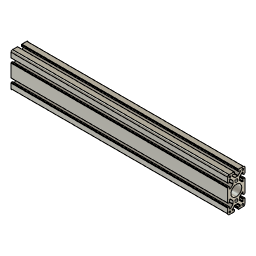
Profile 40x80 (Autodesk Fusion 360 design; units mm, degrees)
Autodesk Fusion 360 part; units mm, degrees
sketch "Sketch1" plane through (0, 0, 0) normal (1, 0, 0) x (0, 1, 0)
  arc A0 (3.0999, -27.5999) -> (3.8071, -27.8928) centre (3.0999, -28.5999) cw
  line L0 (3.8071, -27.8928) -> (9.7071, -33.7929)
  arc A1 (9.7071, -33.7929) -> (9, -35.5) centre (9, -34.5) cw
  line L1 (9, -35.5) -> (5.1, -35.5)
  arc A2 (4.1, -36.5) -> (5.1, -35.5) centre (5.1, -36.5) cw
  line L2 (4.1, -36.5) -> (4.1, -39)
  arc A3 (5.1, -40) -> (4.1, -39) centre (5.1, -39) cw
  line L3 (5.1, -40) -> (16.5, -40)
  arc A4 (20, -36.5) -> (16.5, -40) centre (16.5, -36.5) cw
  line L4 (20, -36.5) -> (20, -25.1)
  arc A5 (19, -24.1) -> (20, -25.1) centre (19, -25.1) cw
  line L5 (19, -24.1) -> (16.5, -24.1)
  arc A6 (15.5, -25.1) -> (16.5, -24.1) centre (16.5, -25.1) cw
  line L6 (15.5, -25.1) -> (15.5, -29)
  arc A7 (15.5, -29) -> (13.7929, -29.7072) centre (14.5, -29) cw
  line L7 (13.7929, -29.7072) -> (7.8929, -23.8071)
  arc A8 (7.8929, -23.8071) -> (7.6, -23.0999) centre (8.6, -23.0999) cw
  circle A9 centre (15, -35) radius 2
  line L8 (0, 0) -> (0, -50) construction
  line L9 (0, 0) -> (50, 0) construction
  arc A10 (0, -12.5) -> (12.5, 0) centre (0, 0) ccw
  line L10 (0, 0) -> (0, -12.5) construction
  line L11 (0, 0) -> (12.5, 0) construction
  arc A11 (0, -23.4) -> (0, -16.6) centre (0, -20) ccw
  line L12 (0, -20) -> (0, -23.4) construction
  line L13 (0, -20) -> (0, -16.6) construction
  line L14 (3.0999, -27.5999) -> (0, -27.5999)
  line L15 (0, -23.4) -> (0, -27.5999)
  line L16 (0, -20) -> (50, -20) construction
  line L17 (7.6, -23.0999) -> (7.6, -20)
  line L18 (0, -16.6) -> (0, -12.5)
  line L19 (15.5, -14.9) -> (15.5, -11)
  arc A12 (20, -14.9) -> (19, -15.9) centre (19, -14.9) cw
  arc A13 (16.5, -15.9) -> (15.5, -14.9) centre (16.5, -14.9) cw
  line L20 (19, -15.9) -> (16.5, -15.9)
  line L21 (7.6, -16.9001) -> (7.6, -20)
  line L22 (13.7929, -10.2928) -> (7.8929, -16.1929)
  arc A14 (7.6, -16.9001) -> (7.8929, -16.1929) centre (8.6, -16.9001) cw
  arc A15 (13.7929, -10.2928) -> (15.5, -11) centre (14.5, -11) cw
  line L23 (20, -14.9) -> (20, 0)
  line L24 (12.5, 0) -> (20, 0)
  line L25 (0, 0) -> (12.5, 0) construction
  arc A16 (9, 35.5) -> (9.7071, 33.7929) centre (9, 34.5) cw
  line L26 (13.7929, 10.2928) -> (7.8929, 16.1929)
  arc A17 (5.1, 35.5) -> (4.1, 36.5) centre (5.1, 36.5) cw
  arc A18 (0, 16.6) -> (0, 23.4) centre (0, 20) ccw
  line L27 (20, 36.5) -> (20, 25.1)
  line L28 (20, 14.9) -> (20, 0)
  arc A19 (20, 25.1) -> (19, 24.1) centre (19, 25.1) cw
  arc A20 (19, 15.9) -> (20, 14.9) centre (19, 14.9) cw
  arc A21 (15.5, 11) -> (13.7929, 10.2928) centre (14.5, 11) cw
  line L29 (0, 20) -> (0, 23.4) construction
  line L30 (9, 35.5) -> (5.1, 35.5)
  arc A22 (4.1, 39) -> (5.1, 40) centre (5.1, 39) cw
  line L31 (0, 23.4) -> (0, 27.5999)
  line L32 (0, 0) -> (0, 12.5) construction
  arc A23 (7.6, 23.0999) -> (7.8929, 23.8071) centre (8.6, 23.0999) cw
  arc A24 (15.5, 14.9) -> (16.5, 15.9) centre (16.5, 14.9) cw
  line L33 (0, 20) -> (0, 16.6) construction
  arc A25 (13.7929, 29.7072) -> (15.5, 29) centre (14.5, 29) cw
  arc A26 (7.8929, 16.1929) -> (7.6, 16.9001) centre (8.6, 16.9001) cw
  line L34 (7.6, 16.9001) -> (7.6, 20)
  line L35 (7.6, 23.0999) -> (7.6, 20)
  line L36 (3.0999, 27.5999) -> (0, 27.5999)
  line L37 (15.5, 25.1) -> (15.5, 29)
  line L38 (3.8071, 27.8928) -> (9.7071, 33.7929)
  arc A27 (16.5, 24.1) -> (15.5, 25.1) centre (16.5, 25.1) cw
  line L39 (4.1, 36.5) -> (4.1, 39)
  line L40 (5.1, 40) -> (16.5, 40)
  arc A28 (3.8071, 27.8928) -> (3.0999, 27.5999) centre (3.0999, 28.5999) cw
  arc A29 (12.5, 0) -> (0, 12.5) centre (0, 0) ccw
  line L41 (15.5, 14.9) -> (15.5, 11)
  line L42 (0, 16.6) -> (0, 12.5)
  line L43 (13.7929, 29.7072) -> (7.8929, 23.8071)
  circle A30 centre (15, 35) radius 2
  line L44 (19, 15.9) -> (16.5, 15.9)
  arc A31 (16.5, 40) -> (20, 36.5) centre (16.5, 36.5) cw
  line L45 (12.5, 0) -> (20, 0)
  line L46 (19, 24.1) -> (16.5, 24.1)
  arc A32 (-19, -15.9) -> (-20, -14.9) centre (-19, -14.9) cw
  line L47 (-9, 35.5) -> (-5.1, 35.5)
  line L48 (-3.0999, 27.5999) -> (0, 27.5999)
  line L49 (-20, 14.9) -> (-20, 0)
  line L50 (-3.8071, 27.8928) -> (-9.7071, 33.7929)
  arc A33 (-4.1, 36.5) -> (-5.1, 35.5) centre (-5.1, 36.5) cw
  line L51 (-7.6, -23.0999) -> (-7.6, -20)
  line L52 (0, 0) -> (-12.5, 0) construction
  arc A34 (-9, -35.5) -> (-9.7071, -33.7929) centre (-9, -34.5) cw
  arc A35 (0, 23.4) -> (0, 16.6) centre (0, 20) ccw
  line L53 (0, 0) -> (0, 12.5) construction
  line L54 (-19, 15.9) -> (-16.5, 15.9)
  line L55 (-13.7929, 10.2928) -> (-7.8929, 16.1929)
  line L56 (-15.5, -25.1) -> (-15.5, -29)
  arc A36 (-7.6, -23.0999) -> (-7.8929, -23.8071) centre (-8.6, -23.0999) cw
  line L57 (-15.5, 14.9) -> (-15.5, 11)
  arc A37 (-19, 24.1) -> (-20, 25.1) centre (-19, 25.1) cw
  arc A38 (-16.5, 15.9) -> (-15.5, 14.9) centre (-16.5, 14.9) cw
  circle A39 centre (-15, -35) radius 2
  line L58 (-12.5, 0) -> (-20, 0)
  line L59 (0, -20) -> (-50, -20) construction
  line L60 (0, 23.4) -> (0, 27.5999)
  line L61 (0, 16.6) -> (0, 12.5)
  arc A40 (-16.5, -40) -> (-20, -36.5) centre (-16.5, -36.5) cw
  line L62 (-19, -15.9) -> (-16.5, -15.9)
  arc A41 (-7.6, 16.9001) -> (-7.8929, 16.1929) centre (-8.6, 16.9001) cw
  line L63 (-7.6, 16.9001) -> (-7.6, 20)
  arc A42 (-20, -25.1) -> (-19, -24.1) centre (-19, -25.1) cw
  line L64 (-20, -36.5) -> (-20, -25.1)
  line L65 (-20, -14.9) -> (-20, 0)
  arc A43 (-7.8929, 23.8071) -> (-7.6, 23.0999) centre (-8.6, 23.0999) cw
  circle A44 centre (-15, 35) radius 2
  arc A45 (-9.7071, 33.7929) -> (-9, 35.5) centre (-9, 34.5) cw
  arc A46 (-5.1, 40) -> (-4.1, 39) centre (-5.1, 39) cw
  line L66 (-19, -24.1) -> (-16.5, -24.1)
  line L67 (-12.5, 0) -> (-20, 0)
  line L68 (0, -20) -> (0, -23.4) construction
  arc A47 (0, -16.6) -> (0, -23.4) centre (0, -20) ccw
  line L69 (0, 20) -> (0, 16.6) construction
  line L70 (0, 20) -> (0, 23.4) construction
  arc A48 (-15.5, 29) -> (-13.7929, 29.7072) centre (-14.5, 29) cw
  arc A49 (-3.0999, 27.5999) -> (-3.8071, 27.8928) centre (-3.0999, 28.5999) cw
  line L71 (0, -23.4) -> (0, -27.5999)
  arc A50 (-4.1, -39) -> (-5.1, -40) centre (-5.1, -39) cw
  line L72 (-4.1, -36.5) -> (-4.1, -39)
  line L73 (-3.8071, -27.8928) -> (-9.7071, -33.7929)
  line L74 (0, -20) -> (0, -16.6) construction
  arc A51 (-12.5, 0) -> (0, -12.5) centre (0, 0) ccw
  line L75 (-13.7929, -10.2928) -> (-7.8929, -16.1929)
  arc A52 (-15.5, -14.9) -> (-16.5, -15.9) centre (-16.5, -14.9) cw
  arc A53 (0, 12.5) -> (-12.5, 0) centre (0, 0) ccw
  arc A54 (-20, 36.5) -> (-16.5, 40) centre (-16.5, 36.5) cw
  line L76 (-4.1, 36.5) -> (-4.1, 39)
  line L77 (-13.7929, 29.7072) -> (-7.8929, 23.8071)
  line L78 (-7.6, 23.0999) -> (-7.6, 20)
  line L79 (0, -16.6) -> (0, -12.5)
  arc A55 (-13.7929, -29.7072) -> (-15.5, -29) centre (-14.5, -29) cw
  line L80 (-9, -35.5) -> (-5.1, -35.5)
  line L81 (-3.0999, -27.5999) -> (0, -27.5999)
  line L82 (-13.7929, -29.7072) -> (-7.8929, -23.8071)
  arc A56 (-5.1, -35.5) -> (-4.1, -36.5) centre (-5.1, -36.5) cw
  arc A57 (-15.5, -11) -> (-13.7929, -10.2928) centre (-14.5, -11) cw
  line L83 (-15.5, -14.9) -> (-15.5, -11)
  arc A58 (-7.8929, -16.1929) -> (-7.6, -16.9001) centre (-8.6, -16.9001) cw
  line L84 (-20, 36.5) -> (-20, 25.1)
  arc A59 (-20, 14.9) -> (-19, 15.9) centre (-19, 14.9) cw
  arc A60 (-15.5, 25.1) -> (-16.5, 24.1) centre (-16.5, 25.1) cw
  line L85 (-19, 24.1) -> (-16.5, 24.1)
  line L86 (-15.5, 25.1) -> (-15.5, 29)
  arc A61 (-13.7929, 10.2928) -> (-15.5, 11) centre (-14.5, 11) cw
  line L87 (-5.1, 40) -> (-16.5, 40)
  line L88 (0, 0) -> (0, -12.5) construction
  arc A62 (-3.8071, -27.8928) -> (-3.0999, -27.5999) centre (-3.0999, -28.5999) cw
  arc A63 (-16.5, -24.1) -> (-15.5, -25.1) centre (-16.5, -25.1) cw
  line L89 (0, 0) -> (-12.5, 0) construction
  line L90 (-7.6, -16.9001) -> (-7.6, -20)
  line L91 (-5.1, -40) -> (-16.5, -40)
  point P0 (0, 20)
  point P1 (0, 20)
  point P2 (-50, 0)
  point P3 (0, -50)
  dimension "d32" = 3.5
  dimension "d35" = 4.5
  dimension "d36" = 1
  dimension "d37" = 1
  dimension "d38" = 1
  dimension "d39" = 1
  dimension "d40" = 4.5
  dimension "d45" = 1
  dimension "d46" = 1
  dimension "d47" = 1
  dimension "d48" = 1
  dimension "d60" = 4
  dimension "d74" = 12.5
  dimension "d75" = 90
  dimension "d76" = 40
  dimension "d77" = 3.4
  dimension "d79" = 20
  dimension "d81" = 35.5
  dimension "d82" = 4.1
  dimension "d83" = 4.1
  dimension "d86" = 20
  dimension "d87" = 7.9
  dimension "d88" = 7.6
  dimension "d90" = 15
  dimension "d91" = 15
  dimension "d92" = 1
  dimension "d93" = 1
  dimension "d94" = 9
  dimension "d95" = 9
  constraint tangent A0 L0
  constraint tangent L0 A1
  constraint tangent L1 A2
  constraint tangent A2 L2
  constraint perpendicular L1 L2
  constraint tangent L2 A3
  constraint tangent A3 L3
  constraint perpendicular L2 L3
  constraint tangent L3 A4
  constraint perpendicular L3 L4
  constraint tangent L4 A5
  constraint tangent A5 L5
  constraint perpendicular L4 L5
  constraint tangent L5 A6
  constraint tangent A6 L6
  constraint perpendicular L5 L6
  constraint tangent L6 A7
  constraint tangent L7 A8
  constraint parallel L0 L7
  constraint equal L0 L7
  constraint vertical L8
  constraint coincident L8.start L9.start
  constraint perpendicular L8 L9
  constraint coincident L8 A11.centre
  constraint coincident L8 L14.end
  constraint tangent A0 L14
  constraint parallel L8 L15
  constraint coincident A11.centre L12.start
  constraint perpendicular L8 L16
  constraint coincident L16 L17.end
  constraint tangent A8 L17
  constraint equal L1 L6
  constraint equal L3 L4
  constraint perpendicular L14 L17
  constraint equal L14 L17
  constraint parallel L8 L17
  constraint parallel L8 L18
  constraint symmetric L4.end L16 A12.start
  constraint symmetric A5.start L16 A12.end
  constraint symmetric A5 L16 A12
  constraint symmetric L5.end L16 A13.start
  constraint symmetric A6.start L16 L19.start
  constraint symmetric A6 L16 A13
  constraint symmetric L6.end L16 L19.end
  constraint symmetric A8.end L16 L21.start
  constraint symmetric A7.end L16 L22.start
  constraint symmetric A7 L16 A15
  constraint symmetric L7.end L16 L22.end
  constraint symmetric A8 L16 A14
  constraint symmetric L16 L17.end L21.end
  constraint coincident L9 L23.end
  constraint tangent A12 L23
  constraint perpendicular L23 L24
  constraint symmetric L8.start L9 A10.centre
  constraint symmetric A0.start L9 L36.start
  constraint symmetric A0.end L9 L38.start
  constraint symmetric A0 L9 A28
  constraint symmetric L0.end L9 A16.end
  constraint symmetric A1.end L9 A16.start
  constraint symmetric A1 L9 A16
  constraint symmetric L1.end L9 A17.start
  constraint symmetric A2.start L9 A17.end
  constraint symmetric A2 L9 A17
  constraint symmetric L2.end L9 A22.start
  constraint symmetric A3.start L9 A22.end
  constraint symmetric A3 L9 A22
  constraint symmetric L3.end L9 L40.end
  constraint symmetric A4.start L9 L27.start
  constraint symmetric A4 L9 A31
  constraint symmetric L4.end L9 L27.end
  constraint symmetric A5.start L9 A19.end
  constraint symmetric A5 L9 A19
  constraint symmetric L5.end L9 A27.start
  constraint symmetric A6.start L9 L37.start
  constraint symmetric A6 L9 A27
  constraint symmetric L6.end L9 A25.end
  constraint symmetric A8.end L9 A23.start
  constraint symmetric A7.end L9 A25.start
  constraint symmetric A7 L9 A25
  constraint symmetric L7.end L9 A23.end
  constraint symmetric A8 L9 A23
  constraint symmetric A9 L9 A30
  constraint symmetric L9 A10.start L32.end
  constraint symmetric L9 A10.end L11.end
  constraint symmetric L9 A10 A29
  constraint symmetric L9 A11.start A18.end
  constraint symmetric L9 A11.end A18.start
  constraint symmetric L9 A11 A18
  constraint symmetric L9 L14.end L31.end
  constraint symmetric L9 A11.centre P1
  constraint symmetric L9 L17.end L34.end
  constraint symmetric L9 L22.end L26.end
  constraint symmetric L9 A13.start A24.end
  constraint symmetric L9 L22.start L26.start
  constraint symmetric L9 L21.start A26.end
  constraint symmetric L9 L19.end A21.start
  constraint symmetric L9 L19.start A24.start
  constraint symmetric L9 A12.start L28.start
  constraint symmetric L9 A12.end A20.start
  constraint symmetric L9 A12 A20
  constraint symmetric L9 A13 A24
  constraint symmetric L9 A14 A26
  constraint symmetric L9 A15 A21
  constraint symmetric L9 L23.end L24.end
  constraint symmetric L9.start L8 A10.centre
  constraint symmetric A0.start L8 L81.start
  constraint symmetric A0.end L8 L73.start
  constraint symmetric A0 L8 A62
  constraint symmetric L0.end L8 A34.end
  constraint symmetric A1.end L8 A34.start
  constraint symmetric A1 L8 A34
  constraint symmetric L1.end L8 L80.end
  constraint symmetric A2.start L8 L72.start
  constraint symmetric A2 L8 A56
  constraint symmetric L2.end L8 A50.start
  constraint symmetric A3.start L8 A50.end
  constraint symmetric A3 L8 A50
  constraint symmetric L3.end L8 A40.start
  constraint symmetric A4.start L8 A40.end
  constraint symmetric A4 L8 A40
  constraint symmetric L4.end L8 A42.start
  constraint symmetric A5.start L8 A42.end
  constraint symmetric A5 L8 A42
  constraint symmetric L5.end L8 L66.end
  constraint symmetric A6.start L8 L56.start
  constraint symmetric A6 L8 A63
  constraint symmetric L6.end L8 L56.end
  constraint symmetric A8.end L8 L51.start
  constraint symmetric A7.end L8 A55.start
  constraint symmetric A7 L8 A55
  constraint symmetric L7.end L8 A36.end
  constraint symmetric A8 L8 A36
  constraint symmetric A9 L8 A39
  constraint symmetric P3 L8 L8.end
  constraint symmetric L8 L9.start A10.centre
  constraint symmetric L8 L9.end P2
  constraint symmetric L8 A10.start L10.end
  constraint symmetric L8 A10.end L52.end
  constraint symmetric L8 A10 A51
  constraint symmetric L8 A11.start L12.end
  constraint symmetric L8 A11.end L13.end
  constraint symmetric L8 A11 A47
  constraint symmetric L8 L14.end L15.end
  constraint symmetric L8 A11.centre L12.start
  constraint symmetric L8 L16.end L59.end
  constraint symmetric L8 L17.end L51.end
  constraint symmetric L8 L22.end L75.end
  constraint symmetric L8 A13.start L62.end
  constraint symmetric L8 L22.start L75.start
  constraint symmetric L8 L21.start A58.end
  constraint symmetric L8 L19.end A57.start
  constraint symmetric L8 L19.start A52.start
  constraint symmetric L8 A12.start A32.end
  constraint symmetric L8 A12.end A32.start
  constraint symmetric L8 A12 A32
  constraint symmetric L8 A13 A52
  constraint symmetric L8 A14 A58
  constraint symmetric L8 A15 A57
  constraint symmetric L8 L23.end L49.end
  constraint symmetric L8 A21.start L57.end
  constraint symmetric L8 L34.end L63.end
  constraint symmetric L8 A19.end A37.start
  constraint symmetric L8 L31.end L36.end
  constraint symmetric L8 L26.end L55.end
  constraint symmetric L8 L27.end A37.end
  constraint symmetric L8 A16.start L47.start
  constraint symmetric L8 L36.start L48.start
  constraint symmetric L8 A17.end A33.start
  constraint symmetric L8 A22.start A46.end
  constraint symmetric L8 L38.start L50.start
  constraint symmetric L8 A23.end A43.start
  constraint symmetric L8 A17.start L47.end
  constraint symmetric L8 L32.end A29.end
  constraint symmetric L8 L28.start L49.start
  constraint symmetric L8 A27.start A60.end
  constraint symmetric L8 L37.start A60.start
  constraint symmetric L8 L26.start L55.start
  constraint symmetric L8 A25.end A48.start
  constraint symmetric L8 L27.start A54.start
  constraint symmetric L8 P1 P0
  constraint symmetric L8 A23.start A43.end
  constraint symmetric L8 L40.end A54.end
  constraint symmetric L8 A20.start L54.start
  constraint symmetric L8 A24.end L54.end
  constraint symmetric L8 A25.start A48.end
  constraint symmetric L8 A18.end L29.end
  constraint symmetric L8 A22.end A46.start
  constraint symmetric L8 A26.end A41.start
  constraint symmetric L8 A24.start L57.start
  constraint symmetric L8 A16.end L50.end
  constraint symmetric L8 A18.start L33.end
  constraint symmetric L8 A16 A45
  constraint symmetric L8 A17 A33
  constraint symmetric L8 A18 A35
  constraint symmetric L8 A19 A37
  constraint symmetric L8 A20 A59
  constraint symmetric L8 A21 A61
  constraint symmetric L8 A22 A46
  constraint symmetric L8 A23 A43
  constraint symmetric L8 A24 A38
  constraint symmetric L8 A25 A48
  constraint symmetric L8 A26 A41
  constraint symmetric L8 A27 A60
  constraint symmetric L8 A28 A49
  constraint symmetric L8 A29 A53
  constraint symmetric L8 A30 A44
  constraint symmetric L8 A31 A54
  measures "d32" radius of A4
  measures "d35" distance of L1.end A3.start
  measures "d36" radius of A3
  measures "d37" radius of A2
  measures "d38" radius of A5
  measures "d39" radius of A6
  measures "d40" distance of L4.end A6.start
  measures "d45" radius of A1
  measures "d46" radius of A7
  measures "d47" radius of A8
  measures "d48" radius of A0
  measures "d60" diameter of A9
  measures "d74" radius of A10
  measures "d75" angle of L10 L11
  measures "d76" vertical distance of A3.start L8.start
  measures "d77" radius of A11
  measures "d79" distance of L8.start A11.centre
  measures "d81" vertical distance of L8.start L1.end
  measures "d82" distance of L2.end L8
  measures "d83" distance of A5.start L16
  measures "d86" horizontal distance of A4.start A11.centre
  measures "d87" horizontal distance of A6.start L17.end
  measures "d88" distance of A11.centre L17.end
  measures "d90" horizontal distance of A9.centre A11.centre
  measures "d91" vertical distance of A9.centre A11.centre
  measures "d92" distance of A7.centre L7
  measures "d93" distance of A1.centre L1
  measures "d94" vertical distance of A7.centre A11.centre
  measures "d95" horizontal distance of A1.centre A11.centre
extrude "Extrude3" add sketch "Sketch1" along normal blind 500 contours A0 L0 A1 L1 A2 L2 A3 L3 A4 L4 A5 L5 A6 L6 A7 L7 A8 A10 A11 L14 L15 L17 L18 L19 A12 A13 L20 L21 L22 A14 A15 L23 L24 L45 L71 L79 | L15 L18 A32 L51 A34 L56 A36 L58 A40 L62 A42 L64 L65 L66 L67 A47 L71 A50 L72 L73 A51 L75 A52 L79 A55 L80 L81 L82 A56 A57 L83 A58 A62 A63 L90 L91 | L24 A16 L26 A17 A18 L27 L28 A19 A20 A21 L30 A22 L31 A23 A24 A25 A26 L34 L35 L36 L37 L38 A27 L39 L40 A28 A29 L41 L42 L43 L44 A31 L45 L46 L60 L61 | L31 L42 L47 L48 L49 L50 A33 A35 L54 L55 L57 A37 A38 L58 L60 L61 A41 L63 A43 A45 A46 L67 A48 A49 A53 A54 L76 L77 L78 L84 A59 A60 L85 L86 A61 L87
equation "Length = 500 mm"
equation "d96 = Length"
named bodies: "Body"
